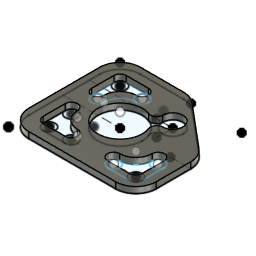
que1 v5 (Autodesk Fusion 360 design; units mm, degrees)
Autodesk Fusion 360 part; units mm, degrees
sketch "Sketch3" plane through (0, 0, 0) normal (0, 0, 1) x (1, 0, 0)
  line L0 (0, 10) -> (0, 45)
  line L1 (10, 55) -> (31.3603, 55)
  line L2 (52.8119, 0) -> (10, 0)
  line L3 (62.8119, 27) -> (52.8119, 27) construction
  line L4 (62.8119, 27) -> (62.8119, 10)
  line L5 (37.7882, 52.6604) -> (59.2397, 34.6604)
  arc A0 (62.8119, 27) -> (59.2397, 34.6604) centre (52.8119, 27) ccw
  arc A1 (37.7882, 52.6604) -> (31.3603, 55) centre (31.3603, 45) ccw
  arc A2 (10, 55) -> (0, 45) centre (10, 45) ccw
  arc A3 (52.8119, 0) -> (62.8119, 10) centre (52.8119, 10) ccw
  arc A4 (0, 10) -> (10, 0) centre (10, 10) ccw
  line L6 (0, 27) -> (28, 27) construction
  line L7 (0, 40) -> (41, 40) construction
  circle A5 centre (41, 40) radius 5
  circle A6 centre (10, 10) radius 3
  circle A7 centre (21, 10) radius 3
  circle A8 centre (10, 21) radius 3
  line L8 (7, 21) -> (7, 10)
  line L9 (10, 7) -> (21, 7)
  arc A9 (13, 21) -> (21, 13) centre (21, 21) ccw
  circle A10 centre (52.8119, 10) radius 3
  circle A11 centre (41.8119, 10) radius 3
  circle A12 centre (52.8119, 21) radius 3
  line L10 (41.8119, 7) -> (52.8119, 7)
  line L11 (55.809, 9.8683) -> (55.8119, 20.9992)
  line L12 (49.8119, 21.0011) -> (49.8119, 20.9971)
  line L13 (41.809, 13) -> (41.8129, 13)
  arc A13 (41.809, 13) -> (49.8119, 20.9971) centre (41.8119, 21) ccw
  circle A14 centre (10, 45) radius 3
  circle A15 centre (21, 45) radius 3
  circle A16 centre (10, 34) radius 3
  line L14 (7, 34) -> (7, 45)
  line L15 (10, 48) -> (21, 48)
  line L16 (21, 42) -> (21, 42)
  arc A17 (21, 42) -> (13, 34) centre (21, 34) ccw
  line L17 (41, 40) -> (41, 32) construction
  line L18 (41, 40) -> (33, 40) construction
  circle A18 centre (28, 27) radius 10.9284
  arc A19 (31.9231, 37.2) -> (36, 40) centre (33, 40) ccw
  arc A20 (41, 35) -> (38.2, 30.9231) centre (41, 32) ccw
  point P0 (0, 55)
  point P1 (60, 55)
  point P2 (35, 55)
  dimension "d35" = 55
  dimension "d36" = 60
  dimension "d37" = 25
  dimension "d39" = 10
  dimension "d40" = 28
  dimension "d41" = 20
  dimension "d42" = 140
  dimension "d43" = 10
  dimension "d44" = 10
  dimension "d45" = 10
  dimension "d46" = 10
  dimension "d51" = 28
  dimension "d52" = 28
  dimension "d53" = 41
  dimension "d54" = 15
  dimension "d55" = 10
  dimension "d56" = 6
  dimension "d57" = 6
  dimension "d58" = 6
  dimension "d60" = 55
  dimension "d62" = 11
  dimension "d63" = 11
  dimension "d64" = 8
  dimension "d65" = 6
  dimension "d66" = 6
  dimension "d67" = 6
  dimension "d68" = 8
  dimension "d69" = 11
  dimension "d70" = 11
  dimension "d71" = 6
  dimension "d72" = 6
  dimension "d73" = 6
  dimension "d74" = 11
  dimension "d75" = 11
  dimension "d76" = 8
  dimension "d79" = 8
  dimension "d80" = 8
  constraint vertical L0
  constraint perpendicular L0 L1
  constraint perpendicular L0 L2
  constraint coincident P1 L1
  constraint coincident L3.end A0.centre
  constraint tangent L4 A0
  constraint tangent L5 A0
  constraint coincident L1 P2
  constraint coincident P2 L5
  constraint tangent L1 A1
  constraint tangent L5 A1
  constraint coincident P0 L0
  constraint coincident P0 L1
  constraint tangent L0 A2
  constraint tangent L1 A2
  constraint tangent L2 A3
  constraint tangent L4 A3
  constraint coincident origin L0
  constraint tangent L0 A4
  constraint tangent L2 A4
  constraint coincident L0 L6.start
  constraint perpendicular L0 L6
  constraint coincident L0 L7.start
  constraint perpendicular L0 L7
  constraint coincident L7.end A5.centre
  constraint concentric A4 A6
  constraint coincident A8 L8.start
  constraint coincident A6 L8.end
  constraint tangent A6 L8
  constraint coincident A6 L9.start
  constraint coincident A7 L9.end
  constraint tangent A7 L9
  constraint tangent A6 L9
  constraint tangent A8 L8
  constraint horizontal L9
  constraint vertical L8
  constraint tangent A8 A9
  constraint tangent A7 A9
  constraint concentric A3 A10
  constraint coincident A11 L10.start
  constraint coincident A10 L10.end
  constraint tangent A10 L10
  constraint coincident A10 L11.start
  constraint coincident A12 L11.end
  constraint tangent A12 L11
  constraint coincident A12 L12.start
  constraint coincident A11 L13.end
  constraint tangent A11 L10
  constraint tangent A12 L12
  constraint tangent A11 L13
  constraint perpendicular L12 L13
  constraint tangent L12 A13
  constraint tangent L13 A13
  constraint concentric A2 A14
  constraint coincident A16 L14.start
  constraint coincident A14 L14.end
  constraint tangent A14 L14
  constraint coincident A14 L15.start
  constraint coincident A15 L15.end
  constraint tangent A15 L15
  constraint horizontal L15
  constraint coincident A15 L16.start
  constraint tangent A15 L16
  constraint tangent A16 L14
  constraint tangent L16 A17
  constraint perpendicular L7 L17
  constraint coincident L17.end A20.centre
  constraint tangent A5 A20
  constraint perpendicular L17 L18
  constraint coincident L18.end A19.centre
  constraint tangent A5 A19
  constraint coincident L6.end A18.centre
  constraint tangent A18 A20
  constraint tangent A18 A19
  constraint coincident L7 A19.end
  constraint coincident A18 A19.start
  constraint coincident A18 A20.end
  constraint coincident A5 A20.start
  measures "d35" distance of origin P0
  measures "d36" distance of P0 P1
  measures "d37" distance of P1 P2
  measures "d39" distance of L3.start L3.end
  measures "d40" distance of L1 L3
  measures "d41" diameter of A0
  measures "d42" angle of L1 L5
  measures "d43" radius of A1
  measures "d44" radius of A2
  measures "d45" radius of A3
  measures "d46" radius of A4
  measures "d51" distance of L6.start L6.end
  measures "d52" distance of L1 L6
  measures "d53" distance of L7.start L7.end
  measures "d54" distance of L1 L7
  measures "d55" diameter of A5
  measures "d56" diameter of A6
  measures "d57" diameter of A7
  measures "d58" diameter of A8
  measures "d60" distance of L1 L2
  measures "d62" distance of A4.centre A7.centre
  measures "d63" distance of A4.centre A8.centre
  measures "d64" radius of A9
  measures "d65" diameter of A10
  measures "d66" diameter of A11
  measures "d67" diameter of A12
  measures "d68" radius of A13
  measures "d69" distance of A3.centre A12.centre
  measures "d70" distance of A3.centre A11.centre
  measures "d71" diameter of A14
  measures "d72" diameter of A15
  measures "d73" diameter of A16
  measures "d74" vertical distance of L14.start L14.end
  measures "d75" distance of L15.start L15.end
  measures "d76" radius of A17
  measures "d79" distance of L7.end L18.end
  measures "d80" distance of L7.end L17.end
extrude "Extrude3" add sketch "Sketch3" along normal blind 3
